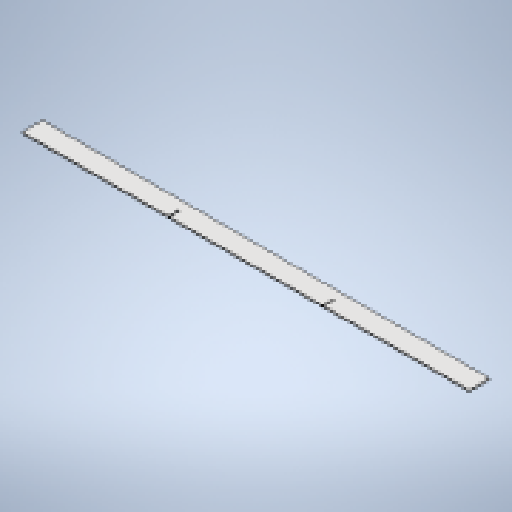
# Autodesk Inventor part: MSC 108 rib cone
Saved by Autodesk Inventor 2025 (Build 290162010, 162A)
## iProperties
Created: 2024-06-26
Part Number: MSC 108 rib cone
Material: Stainless Steel
Document SubType Name: Sheet Metal
Designer: pokla
Density: 8 g/cm^3
Sheet Metal Rule: AISI304 3mm Die 32
Appearance: Default
Stock Number: МОО 108 шпангоут конус
Author: pokla
Autodesk Inventor part; units mm, degrees
ref_plane "YZ Plane" through (0, 0, 0) normal (1, 0, 0) x (0, 1, 0)
ref_plane "XZ Plane" through (0, 0, 0) normal (0, 1, 0) x (-1, 0, 0)
ref_plane "XY Plane" through (0, 0, 0) normal (0, 0, 1) x (1, 0, 0)
sketch "Sketch1" plane through (0, 0, 0) normal (0, 0, 1) x (1, 0, 0)
  line L0 (-600, 50) -> (600, 50)
  line L1 (600, 50) -> (600, 0)
  line L2 (600, 0) -> (-600, 0)
  line L3 (-600, 0) -> (-600, 50)
  circle A0 centre (-600, 0) radius 25
  circle A1 centre (600, 0) radius 25
  line L4 (600, 0) -> (657.2042, 48)
  line L5 (657.2042, 48) -> (657.2042, 50)
  line L6 (657.2042, 50) -> (600, 50)
  point P0 (0, 0)
  point P1 (0, 0)
  point P2 (-600, 25)
  point P3 (-575, 0)
  point P4 (575, 0)
  point P5 (600, 25)
  point P6 (619.1511, 16.0697)
  dimension "d16" = 50
  dimension "d17" = 1200
  dimension "d18" = 50
  dimension "d19" = 50
  dimension "d32" = 2
  dimension "d33" = 50
  measures "d16" distance of L0.end L1.end
  measures "d17" distance of L0.start L0.end
  measures "d18" diameter of A0
  measures "d19" diameter of A1
  measures "d32" distance of L4.end L5.end
  measures "d33" angle of L1 L4
extrude "Plate2" add sketch "Sketch1" against normal blind 3 contours L0 L1 A1 L2 A0 L3 | A0 L2 L3 | L1 L2 A1 picked at (-598.1457, 16.4577)
sketch "Sketch2" plane through (0, 0, 0) normal (0, 0, 1) x (1, 0, 0)
  line L0 (-600, 0) -> (600, 0) projected
  line L1 (190, 0) -> (190, 50) construction
  line L2 (600, 50) -> (-600, 50) projected
  line L3 (188.5, 26) -> (191.5, 26)
  line L4 (191.5, 26) -> (191.5, 0)
  line L5 (191.5, 0) -> (188.5, 0)
  line L6 (188.5, 0) -> (188.5, 26)
  line L7 (-190, 50) -> (-190, 0) construction
  line L8 (-191.5, 26) -> (-188.5, 26)
  line L9 (-188.5, 26) -> (-188.5, 0)
  line L10 (-188.5, 0) -> (-191.5, 0)
  line L11 (-191.5, 0) -> (-191.5, 26)
  point P0 (0, 0)
  point P1 (0, 0)
  point P2 (188.5, 0)
  point P3 (0, 0)
  point P4 (-191.5, 0)
  point P5 (-188.5, 0)
  dimension "d21" = 190
  dimension "d22" = 3
  dimension "d23" = 26
  dimension "d29" = 190
  dimension "d30" = 3
  dimension "d31" = 26
  constraints: 20 end point, 4 midpoint, 4 parallel, 4 point on line, 3 perpendicular, 2 horizontal, 1 vertical
  measures "d21" distance from line of point (0, 0) L1
  measures "d22" distance of L4.end L5.end
  measures "d23" distance of L3.end L4.end
  measures "d29" distance from line of point (0, 0) L7
  measures "d30" distance of L9.end L10.end
  measures "d31" distance of L8.end L9.end
extrude "Extrusion1" cut sketch "Sketch2" against normal through all
sketch "Sketch3" plane through (0, 0, -3) normal (0, 0, -1) x (-1, 0, 0)
  line L0 (-191.5, 0) -> (-191.5, 26) projected
  line L1 (-191.5, 26) -> (-188.5, 26) projected
  line L2 (-188.5, 26) -> (-188.5, 0) projected
  line L3 (188.5, 0) -> (-188.5, 0) projected
  line L4 (188.5, 0) -> (188.5, 26) projected
  line L5 (188.5, 26) -> (191.5, 26) projected
  line L6 (191.5, 26) -> (191.5, 0) projected
  line L7 (600, 0) -> (191.5, 0) projected
  line L8 (600, 50) -> (600, 0) projected
  line L9 (-600, 50) -> (600, 50) projected
  line L10 (-600, 0) -> (-600, 50) projected
  line L11 (-191.5, 0) -> (-600, 0) projected
  line L12 (600, 0) -> (191.5, 0) projected
  line L13 (550, 0) -> (550, 50)
  line L14 (-550, 0) -> (-550, 50)
  point P0 (0, 0)
  dimension "d34" = 50
  dimension "d35" = 50
  constraints: 4 end point, 4 point on line, 2 vertical
  measures "d34" distance between parallel lines of L10 L14
  measures "d35" distance between parallel lines of L8 L13
extrude "Extrusion2" cut sketch "Sketch3" against normal through all contours L11 L10 L9 L14 | L9 L8 L7 L13
equation "\"d22\" = Thickness"
equation "\"d29\" = d21"
equation "\"d30\" = Thickness"
equation "\"d31\" = d23"
equation "\"d35\" = d34"
equation "\"d20\" = Thickness"
equation "\"BendReliefWidth\" = Thickness"
equation "\"BendReliefDepth\" = 0.5 * Thickness"
equation "\"CornerReliefSize\" = 4 * Thickness"
equation "\"MinimumRemnant\" = 2 * Thickness"
equation "\"TransitionRadius\" = BendRadius"
equation "\"JacobiRadiusSize\" = BendRadius"
equation "\"GapSize\" = Thickness"
equation "\"Thickness\" = 3"
equation "\"BendRadius\" = 5"
body "Solid2"
